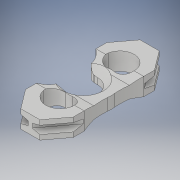
# Autodesk Inventor part: Attempted redesign Andrew.8.Offcentered.LargerAccesss
Saved by Autodesk Inventor 2017 (Build 210142000, 142)
## iProperties
Created: 2016-03-15
Part Number: Attempted redesign Andrew.8.Offcentered.LargerAccesss
Material: Generic
Document SubType Name: Modeling
Designer: Opto Neuro Core
Density: 1 g/cm^3
Appearance: Default
Author: Opto Neuro Core
Autodesk Inventor part; units mm, degrees
ref_plane "YZ Plane" through (0, 0, 0) normal (1, 0, 0) x (0, 1, 0)
ref_plane "XZ Plane" through (0, 0, 0) normal (0, 1, 0) x (-1, 0, 0)
ref_plane "XY Plane" through (0, 0, 0) normal (0, 0, 1) x (1, 0, 0)
sketch "Sketch1" plane through (0, 0, 0) normal (0, 1, 0) x (-1, 0, 0)
  line L0 (0.0095, 15.8699) -> (12.7095, 15.8699) construction
  line L1 (8.8995, 15.8699) -> (12.7095, 10.7899) construction
  line L2 (3.8195, 15.8699) -> (0.0095, 10.7899) construction
  line L3 (8.8995, 15.8699) -> (3.8195, 15.8699) construction
  line L4 (0.0095, 10.7899) -> (0.0095, 7.9324) construction
  line L5 (12.7095, 10.7899) -> (12.7095, 7.9324) construction
  line L6 (12.7095, 7.9324) -> (0.0095, 7.9324) construction
  line L7 (12.7095, 7.9324) -> (0.0095, 7.9324)
  line L8 (0.0095, 7.9324) -> (0.0095, 10.7899)
  line L9 (0.0095, 10.7899) -> (3.8195, 15.8699)
  line L10 (3.8195, 15.8699) -> (8.8995, 15.8699)
  line L11 (8.8995, 15.8699) -> (12.7095, 10.7899)
  line L12 (12.7095, 10.7899) -> (12.7095, 7.9324)
  line L13 (6.3547, -0.0026) -> (-13.1747, -0.0026) construction
  line L14 (0.0095, -15.875) -> (12.7095, -15.875) construction
  line L15 (8.8995, -15.875) -> (12.7095, -10.795) construction
  line L16 (3.8195, -15.875) -> (0.0095, -10.795) construction
  line L17 (8.8995, -15.875) -> (3.8195, -15.875) construction
  line L18 (0.0095, -10.795) -> (0.0095, -7.9375) construction
  line L19 (12.7095, -10.795) -> (12.7095, -7.9375) construction
  line L20 (12.7095, -7.9375) -> (0.0095, -7.9375) construction
  line L21 (12.7095, -7.9375) -> (0.0095, -7.9375)
  line L22 (0.0095, -7.9375) -> (0.0095, -10.795)
  line L23 (0.0095, -10.795) -> (3.8195, -15.875)
  line L24 (3.8195, -15.875) -> (8.8995, -15.875)
  line L25 (8.8995, -15.875) -> (12.7095, -10.795)
  line L26 (12.7095, -10.795) -> (12.7095, -7.9375)
  point P0 (0, 0)
  dimension "d8" = 6.35
  dimension "d83" = 2.8575
  constraints: 54 end point, 8 symmetric about line, 5 collinear, 4 point on line, 3 horizontal, 2 vertical, 1 perpendicular
  measures "d8" distance of L2.start L2.end
  measures "d83" distance of L2.end L4.end
extrude "Extrusion11" add sketch "Sketch1" along normal blind 0.508
sketch "Sketch12" plane through (0, 0.508, 0) normal (0, 1, 0) x (1, 0, 0)
  line L0 (-0.0095, 10.795) -> (-3.8195, 15.875) projected
  line L1 (-3.8195, 15.875) -> (-8.8995, 15.875) projected
  line L2 (-8.8995, 15.875) -> (-12.7095, 10.795) projected
  line L3 (-12.7095, 10.795) -> (-12.7095, 7.9375) projected
  line L4 (-12.7095, 7.9375) -> (-0.0095, 7.9375) projected
  line L5 (-0.0095, 7.9375) -> (-0.0095, 10.795) projected
  line L6 (-3.8195, -15.8699) -> (-0.0095, -10.7899) projected
  line L7 (-0.0095, -10.7899) -> (-0.0095, -7.9324) projected
  line L8 (-0.0095, -7.9324) -> (-12.7095, -7.9324) projected
  line L9 (-12.7095, -7.9324) -> (-12.7095, -10.7899) projected
  line L10 (-12.7095, -10.7899) -> (-8.8995, -15.8699) projected
  line L11 (-8.8995, -15.8699) -> (-3.8195, -15.8699) projected
  point P0 (0, 0)
extrude "Extrusion12" add sketch "Sketch12" along normal blind 0.5207
chamfer "Chamfer17" distance 1.5935 distance2 0.5207 1 edges at (-1.9145, 1.0287, -13.335) measured on face at (-2.3145, 1.0287, -13.035)
chamfer "Chamfer18" distance 1.5935 distance2 0.5207 1 edges at (-10.8045, 1.0287, -13.335) measured on face at (-10.4045, 1.0287, -13.035)
chamfer "Chamfer19" distance 1.5935 distance2 0.5207 1 edges at (-1.9145, 1.0287, 13.3299) measured on face at (-2.3145, 1.0287, 13.0299)
chamfer "Chamfer20" distance 1.5935 distance2 0.5207 1 edges at (-10.8045, 1.0287, 13.3299) measured on face at (-10.4045, 1.0287, 13.0299)
sketch "Sketch14" plane through (0, 1.0287, 0) normal (0, 1, 0) x (1, 0, 0)
  line L0 (-12.7095, 8.1392) -> (-6.9076, 15.875) projected
  line L1 (-12.7095, 8.1392) -> (-12.7095, 7.9375) projected
  line L2 (-12.7095, 7.9375) -> (-0.0095, 7.9375) projected
  line L3 (-0.0095, 7.9375) -> (-0.0095, 8.1392) projected
  line L4 (-5.8113, 15.875) -> (-0.0095, 8.1392) projected
  line L5 (-5.8113, 15.875) -> (-6.9076, 15.875) projected
  line L6 (-6.9076, -15.8699) -> (-12.7095, -8.1341) projected
  line L7 (-6.9076, -15.8699) -> (-5.8113, -15.8699) projected
  line L8 (-0.0095, -8.1341) -> (-5.8113, -15.8699) projected
  line L9 (-0.0095, -8.1341) -> (-0.0095, -7.9324) projected
  line L10 (-0.0095, -7.9324) -> (-12.7095, -7.9324) projected
  line L11 (-12.7095, -7.9324) -> (-12.7095, -8.1341) projected
  point P0 (0, 0)
extrude "Extrusion13" add sketch "Sketch14" along normal blind 1.1176
sketch "Sketch15" plane through (0, 2.1463, 0) normal (0, 1, 0) x (1, 0, 0)
  line L0 (-3.8195, 15.875) -> (-0.0095, 10.795) projected
  line L1 (-0.0095, 10.795) -> (-0.0095, 7.9375) projected
  line L2 (-0.0095, 7.9375) -> (-12.7095, 7.9375) projected
  line L3 (-12.7095, 7.9375) -> (-12.7095, 10.795) projected
  line L4 (-12.7095, 10.795) -> (-8.8995, 15.875) projected
  line L5 (-8.8995, 15.875) -> (-3.8195, 15.875) projected
  line L6 (-3.8195, -15.8699) -> (-0.0095, -10.7899) projected
  line L7 (-8.8995, -15.8699) -> (-3.8195, -15.8699) projected
  line L8 (-12.7095, -10.7899) -> (-8.8995, -15.8699) projected
  line L9 (-12.7095, -7.9324) -> (-12.7095, -10.7899) projected
  line L10 (-0.0095, -7.9324) -> (-12.7095, -7.9324) projected
  line L11 (-0.0095, -10.7899) -> (-0.0095, -7.9324) projected
  point P0 (0, 0)
extrude "Extrusion14" add sketch "Sketch15" along normal blind 0.5207
sketch "Sketch16" plane through (0, 2.667, 0) normal (0, 1, 0) x (1, 0, 0)
  line L0 (-0.0095, 10.795) -> (-3.8195, 15.875) projected
  line L1 (-3.8195, 15.875) -> (-8.8995, 15.875) projected
  line L2 (-8.8995, 15.875) -> (-12.7095, 10.795) projected
  line L3 (-12.7095, 10.795) -> (-12.7095, 7.9375) projected
  line L4 (-12.7095, 7.9375) -> (-0.0095, 7.9375) projected
  line L5 (-0.0095, 7.9375) -> (-0.0095, 10.795) projected
  line L6 (-3.8195, -15.8699) -> (-0.0095, -10.7899) projected
  line L7 (-0.0095, -10.7899) -> (-0.0095, -7.9324) projected
  line L8 (-0.0095, -7.9324) -> (-12.7095, -7.9324) projected
  line L9 (-12.7095, -7.9324) -> (-12.7095, -10.7899) projected
  line L10 (-12.7095, -10.7899) -> (-8.8995, -15.8699) projected
  line L11 (-8.8995, -15.8699) -> (-3.8195, -15.8699) projected
  point P0 (0, 0)
extrude "Extrusion15" add sketch "Sketch16" along normal blind 0.508
chamfer "Chamfer21" distance 1.5935 distance2 0.5207 1 edges at (-1.9145, 2.1463, -13.335) measured on face at (-2.3145, 2.1463, -13.035)
chamfer "Chamfer22" distance 1.5935 distance2 0.5207 1 edges at (-10.8045, 2.1463, -13.335) measured on face at (-10.4045, 2.1463, -13.035)
chamfer "Chamfer23" distance 1.5935 distance2 0.5207 1 edges at (-1.9145, 2.1463, 13.3299) measured on face at (-2.3145, 2.1463, 13.0299)
chamfer "Chamfer24" distance 1.5935 distance2 0.5207 1 edges at (-10.8045, 2.1463, 13.3299) measured on face at (-10.4045, 2.1463, 13.0299)
sketch "Sketch18" plane through (0, 3.175, 0) normal (0, 1, 0) x (1, 0, 0)
  line L0 (-0.0095, 10.795) -> (-3.8195, 15.875) construction
  line L1 (-3.8195, 15.875) -> (-8.8995, 15.875) construction
  line L2 (-8.8995, 15.875) -> (-12.7095, 10.795) construction
  line L3 (-12.7095, 10.795) -> (-12.7095, 7.9375) construction
  line L4 (-12.7095, 7.9375) -> (-0.0095, 7.9375) construction
  line L5 (-0.0095, 7.9375) -> (-0.0095, 10.795) construction
  line L6 (-3.8195, -15.8699) -> (-0.0095, -10.7899) construction
  line L7 (-0.0095, -10.7899) -> (-0.0095, -7.9324) construction
  line L8 (-0.0095, -7.9324) -> (-12.7095, -7.9324) construction
  line L9 (-12.7095, -7.9324) -> (-12.7095, -10.7899) construction
  line L10 (-12.7095, -10.7899) -> (-8.8995, -15.8699) construction
  line L11 (-8.8995, -15.8699) -> (-3.8195, -15.8699) construction
  line L12 (-0.0095, 7.9375) -> (-12.7095, 7.9375) construction
  line L13 (-6.3595, 7.9375) -> (-6.3595, -7.9324) construction
  line L14 (-0.0095, 7.9375) -> (-0.0095, -7.9324) construction
  line L15 (-12.7095, 7.9375) -> (-12.7095, -7.9324) construction
  line L16 (-12.7095, 7.9375) -> (-12.7095, 10.795) construction
  line L17 (-0.0095, 9.3663) -> (-4.4274, 3.2863) construction
  line L18 (-4.4274, -3.2812) -> (-0.0095, -9.3611) construction
  line L19 (-0.0095, -10.7899) -> (-0.0095, -7.9324) construction
  line L20 (-12.7095, -8.1341) -> (-12.7095, -10.7899) construction
  line L21 (-12.7095, -9.462) -> (-8.2916, -3.2812) construction
  line L22 (-12.7095, 9.3662) -> (-8.2916, 3.2863) construction
  line L23 (-2.5495, -5.8656) -> (-2.5495, 0.0026) construction
  line L24 (-2.5495, 0.0026) -> (-2.5495, 5.8707) construction
  line L25 (-10.1695, 0.0026) -> (-10.1695, -5.9084) construction
  line L26 (-10.1695, 0.0026) -> (-10.1695, 5.8707) construction
  circle A0 centre (-6.3595, 0.0026) radius 5.715 construction
  line L27 (-0.0095, 7.9375) -> (-3.3041, 4.8322)
  line L28 (-3.3041, -4.8271) -> (-0.0095, -7.9324)
  arc A1 (-3.3041, -4.8271) -> (-3.3041, 4.8322) centre (-6.3595, 0.0026) ccw
  line L29 (-0.0095, 7.9375) -> (-12.7095, 7.9375)
  line L30 (-0.0095, -7.9324) -> (-12.7095, -7.9324)
  circle A2 centre (-9.1475, 0.0122) radius 3.81
  line L31 (11.1379, 29.9505) -> (12.3599, 29.9505)
  line L32 (-12.7095, 7.9375) -> (-12.7095, 1.3643)
  line L33 (-12.7095, -1.3399) -> (-12.7095, 1.3643)
  line L34 (-12.7095, -1.3399) -> (-12.7095, -7.9324)
  point P0 (-9.4149, 4.8322)
  point P1 (-9.4023, -4.8351)
  dimension "d119" = 11.43
  dimension "d162" = 7.62
  constraints: 38 end point, 11 point on line, 8 point on circle, 6 midpoint, 3 centre point, 3 horizontal, 2 collinear, 2 concentric, 2 parallel, 2 vertical
  measures "d119" diameter of A0
  measures "d162" diameter of A2
extrude "Extrusion16" add sketch "Sketch18" against normal blind 3.175 contours L27 A1 L28 L30 L34 A2 L32 L29
fillet "Fillet1" radius 3.175 2 edges at (-3.3041, 1.5875, 4.8271) (-3.3041, 1.5875, -4.8322)
sketch "Sketch19" plane through (0, 3.175, 0) normal (0, 1, 0) x (1, 0, 0)
  arc A0 (-1.5083, -3.0185) -> (-1.5083, 3.0237) centre (-6.3595, 0.0026) ccw construction
  line L0 (-3.8195, 15.875) -> (-8.8995, 15.875) construction
  arc A1 (-11.2107, 3.0237) -> (-11.2092, -3.0209) centre (-6.3595, 0.0026) ccw construction
  line L1 (-12.7095, 8.1392) -> (-6.9076, 15.875) construction
  line L2 (-6.9076, 15.875) -> (-12.7095, 8.1392) construction
  line L3 (-5.8113, 15.875) -> (-0.0095, 8.1392) construction
  line L4 (-0.0095, 8.1392) -> (-5.8113, 15.875) construction
  line L5 (-6.9076, -15.8699) -> (-12.7095, -8.1341) construction
  line L6 (-12.7095, -8.1341) -> (-6.9076, -15.8699) construction
  line L7 (-0.0095, -8.1341) -> (-5.8113, -15.8699) construction
  line L8 (-5.8113, -15.8699) -> (-0.0095, -8.1341) construction
  line L9 (-8.8995, 15.875) -> (-3.8195, 15.875) construction
  line L10 (-8.8995, -15.8699) -> (-3.8195, -15.8699) construction
  line L11 (-6.3595, 15.875) -> (-6.3595, -15.8699) construction
  line L12 (-6.3595, 0.0026) -> (-6.3595, 15.875) construction
  line L13 (-6.3595, 0.0026) -> (-6.3595, -15.8699) construction
  line L14 (-6.3595, -7.9337) -> (5.5565, -7.9337) construction
  line L15 (-6.3595, 7.9388) -> (8.721, 7.9388) construction
  arc A2 (-3.803, 5.1139) -> (-8.916, 5.1139) centre (-6.3595, 7.9388) ccw construction
  arc A3 (-8.916, -5.1087) -> (-3.803, -5.1087) centre (-6.3595, -7.9337) ccw construction
  circle A4 centre (-6.3595, 0.0026) radius 5.715 construction
  arc A5 (-3.803, 5.1139) -> (-8.916, 5.1139) centre (-6.3595, 7.9388) ccw
  arc A6 (-3.803, 5.1139) -> (-8.916, 5.1139) centre (-6.3595, 0.0026) ccw
  arc A7 (-8.916, -5.1087) -> (-3.803, -5.1087) centre (-6.3595, -7.9337) ccw
  arc A8 (-8.916, -5.1087) -> (-3.803, -5.1087) centre (-6.3595, 0.0026) ccw
  point P0 (0, 0)
  dimension "d123" = 7.62
  dimension "d124" = 7.62
  constraints: 16 point on circle, 10 end point, 7 centre point, 4 concentric, 4 midpoint, 3 coincident, 2 horizontal, 1 collinear, 1 perpendicular
  measures "d123" diameter of A2
  measures "d124" diameter of A3
extrude "Extrusion17" cut sketch "Sketch19" against normal blind 25.4
fillet "Fillet2" radius 2.54 4 edges at (-8.916, 1.5875, 5.1087) (-3.803, 1.5875, 5.1087) (-3.803, 1.5875, -5.1139) (-8.916, 1.5875, -5.1139)
sketch "Sketch20" plane through (0, 3.175, 0) normal (0, 1, 0) x (1, 0, 0)
  line L0 (-3.8195, -15.8699) -> (-0.0095, -10.7899) projected
  line L1 (-0.0095, -10.7899) -> (-0.0095, -7.9324) projected
  line L2 (-0.0095, -7.9324) -> (-0.9909, -7.0074) projected
  arc A0 (-1.5083, -3.0185) -> (-0.9909, -7.0074) centre (1.1868, -4.6969) ccw projected
  arc A1 (-1.5083, -3.0185) -> (-1.5083, 3.0237) centre (-6.3595, 0.0026) ccw projected
  arc A2 (-0.9909, 7.0125) -> (-1.5083, 3.0237) centre (1.1868, 4.7021) ccw projected
  line L3 (-0.9909, 7.0125) -> (-0.0095, 7.9375) projected
  line L4 (-0.0095, 7.9375) -> (-0.0095, 10.795) projected
  line L5 (-0.0095, 10.795) -> (-3.8195, 15.875) projected
  line L6 (-3.8195, 15.875) -> (-8.8995, 15.875) projected
  line L7 (-8.8995, 15.875) -> (-12.7095, 10.795) projected
  line L8 (-12.7095, 10.795) -> (-12.7095, 7.9375) projected
  line L9 (-12.7095, 7.9375) -> (-11.7281, 7.0125) projected
  arc A3 (-11.2107, 3.0237) -> (-11.7281, 7.0125) centre (-13.9058, 4.7021) ccw projected
  arc A4 (-11.2107, 3.0237) -> (-11.2092, -3.0209) centre (-6.3595, 0.0026) ccw projected
  arc A5 (-11.7332, -7.018) -> (-11.2092, -3.0209) centre (-13.9035, -4.7006) ccw projected
  line L10 (-11.7332, -7.018) -> (-12.7095, -7.9324) projected
  line L11 (-12.7095, -7.9324) -> (-12.7095, -10.7899) projected
  line L12 (-12.7095, -10.7899) -> (-8.8995, -15.8699) projected
  line L13 (-8.8995, -15.8699) -> (-3.8195, -15.8699) projected
  arc A6 (-7.225, -5.6465) -> (-5.494, -5.6465) centre (-6.3595, 0.0026) ccw projected
  arc A7 (-2.609, -8.6044) -> (-5.494, -5.6465) centre (-5.1093, -8.1572) ccw projected
  arc A8 (-10.11, -8.6044) -> (-2.609, -8.6044) centre (-6.3595, -7.9337) ccw projected
  arc A9 (-7.225, -5.6465) -> (-10.11, -8.6044) centre (-7.6097, -8.1572) ccw projected
  arc A10 (-5.494, 5.6516) -> (-7.225, 5.6516) centre (-6.3595, 0.0026) ccw projected
  arc A11 (-10.11, 8.6095) -> (-7.225, 5.6516) centre (-7.6097, 8.1624) ccw projected
  arc A12 (-2.609, 8.6095) -> (-10.11, 8.6095) centre (-6.3595, 7.9388) ccw projected
  arc A13 (-5.494, 5.6516) -> (-2.609, 8.6095) centre (-5.1093, 8.1624) ccw projected
  circle A14 centre (-6.3595, 0.0026) radius 4.7244 projected
  point P0 (0, 0)
  point P1 (-10.1695, -7.9324)
  point P2 (-2.5495, -7.9324)
  point P3 (-2.5495, 7.9375)
  point P4 (-10.1695, 7.9375)
extrude "Extrusion18" add sketch "Sketch20" along normal blind 0.762
sketch "Sketch21" plane through (0, 0, 0) normal (0, -1, 0) x (1, 0, 0)
  arc A0 (-7.225, -5.6516) -> (-5.494, -5.6516) centre (-6.3595, -0.0026) ccw projected
  arc A1 (-2.609, -8.6095) -> (-5.494, -5.6516) centre (-5.1093, -8.1624) ccw projected
  arc A2 (-10.11, -8.6095) -> (-2.609, -8.6095) centre (-6.3595, -7.9388) ccw projected
  arc A3 (-7.225, -5.6516) -> (-10.11, -8.6095) centre (-7.6097, -8.1624) ccw projected
  arc A4 (-5.494, 5.6465) -> (-7.225, 5.6465) centre (-6.3595, -0.0026) ccw projected
  arc A5 (-10.11, 8.6044) -> (-7.225, 5.6465) centre (-7.6097, 8.1572) ccw projected
  arc A6 (-2.609, 8.6044) -> (-10.11, 8.6044) centre (-6.3595, 7.9337) ccw projected
  arc A7 (-5.494, 5.6465) -> (-2.609, 8.6044) centre (-5.1093, 8.1572) ccw projected
  circle A8 centre (-6.3595, -0.0026) radius 3.81 projected
  line L0 (-3.8195, 15.8699) -> (-0.0095, 10.7899) projected
  line L1 (-8.8995, 15.8699) -> (-3.8195, 15.8699) projected
  line L2 (-12.7095, 10.7899) -> (-8.8995, 15.8699) projected
  line L3 (-12.7095, 7.9324) -> (-12.7095, 10.7899) projected
  line L4 (-12.7095, 7.9324) -> (-11.7332, 7.018) projected
  arc A9 (-11.2092, 3.0209) -> (-11.7332, 7.018) centre (-13.9035, 4.7006) ccw projected
  arc A10 (-11.2092, 3.0209) -> (-11.2107, -3.0237) centre (-6.3595, -0.0026) ccw projected
  arc A11 (-11.7281, -7.0125) -> (-11.2107, -3.0237) centre (-13.9058, -4.7021) ccw projected
  line L5 (-11.7281, -7.0125) -> (-12.7095, -7.9375) projected
  line L6 (-12.7095, -7.9375) -> (-12.7095, -10.795) projected
  line L7 (-12.7095, -10.795) -> (-8.8995, -15.875) projected
  line L8 (-8.8995, -15.875) -> (-3.8195, -15.875) projected
  line L9 (-3.8195, -15.875) -> (-0.0095, -10.795) projected
  line L10 (-0.0095, -10.795) -> (-0.0095, -7.9375) projected
  line L11 (-0.0095, -7.9375) -> (-0.9909, -7.0125) projected
  arc A12 (-1.5083, -3.0237) -> (-0.9909, -7.0125) centre (1.1868, -4.7021) ccw projected
  arc A13 (-1.5083, -3.0237) -> (-1.5083, 3.0185) centre (-6.3595, -0.0026) ccw projected
  arc A14 (-0.9909, 7.0074) -> (-1.5083, 3.0185) centre (1.1868, 4.6969) ccw projected
  line L12 (-0.9909, 7.0074) -> (-0.0095, 7.9324) projected
  line L13 (-0.0095, 10.7899) -> (-0.0095, 7.9324) projected
  point P0 (0, 0)
  point P1 (-10.1695, -7.9375)
  point P2 (-2.5495, -7.9375)
  point P3 (-2.5495, 7.9324)
  point P4 (-10.1695, 7.9324)
extrude "Extrusion19" add sketch "Sketch21" along normal blind 0.762
sketch "Sketch24" plane through (-12.7095, 1.0287, -8.1392) normal (-1, 0, 0) x (0, 0, 1)
  line L0 (0.2017, 2.9083) -> (0.2017, -1.7907) construction
  line L1 (18.9291, 1.6383) -> (16.2733, 1.1176) construction
  line L2 (18.9291, 1.6383) -> (18.9291, 2.9083) construction
  line L3 (16.0716, 2.9083) -> (18.9291, 2.9083) construction
  line L4 (16.0716, 2.1463) -> (16.0716, 2.9083) construction
  line L5 (18.9291, -1.7907) -> (16.0716, -1.7907) construction
  line L6 (18.9291, -1.7907) -> (18.9291, -0.5207) construction
  line L7 (16.2733, 0) -> (18.9291, -0.5207) construction
  line L8 (16.2733, 0) -> (16.2733, 1.1176) construction
  line L9 (3.4122, 2.9083) -> (12.861, 2.9083) construction
  line L10 (5.1155, -1.7907) -> (1.1267, -1.7907) construction
  line L11 (3.4122, -1.7907) -> (3.4122, -1.0287) construction
  line L12 (3.4122, -1.7907) -> (4.1742, -1.7907) construction
  line L13 (12.861, -1.7907) -> (12.861, -1.0287) construction
  line L14 (12.861, -1.7907) -> (13.623, -1.7907) construction
  line L15 (12.861, 2.1463) -> (16.0716, 2.9083)
  line L16 (16.0716, 2.9083) -> (0.2017, 2.9083)
  line L17 (0.2017, 2.9083) -> (0.2017, -1.7907) projected
  line L18 (0.2017, -1.7907) -> (3.4122, -1.0287)
  line L19 (3.4122, -1.0287) -> (12.861, -1.0287)
  line L20 (12.861, -1.0287) -> (16.0716, -1.7907)
  line L21 (16.0716, -1.7907) -> (16.0716, 2.9083) projected
  line L22 (16.0716, -1.7907) -> (0.2017, -1.7907)
  line L23 (12.861, 2.1463) -> (3.4122, 2.1463) projected
  line L24 (3.4122, 2.1463) -> (0.2017, 2.9083)
  line L25 (12.861, 2.1463) -> (3.4122, 2.1463)
  line L26 (16.0716, -1.0287) -> (16.0716, -1.7907) projected
  line L27 (9.4791, 2.1463) -> (16.0716, 2.1463) projected
  line L28 (9.4791, 2.1463) -> (9.4791, -1.0287) projected
  line L29 (16.0716, -1.0287) -> (9.4791, -1.0287) projected
  point P0 (8.1392, -1.0287)
  dimension "d150" = 0.762
  dimension "d151" = 90
  dimension "d152" = 0.762
  dimension "d153" = 90
  constraints: 24 end point, 6 perpendicular, 2 horizontal, 1 parallel, 1 point on line, 1 vertical
  measures "d150" distance of L11.start L11.end
  measures "d151" angle of L12 L11
  measures "d152" distance of L13.start L13.end
  measures "d153" angle of L14 L13
extrude "Extrusion22" cut sketch "Sketch24" against normal through all contours L23 L24 L16 L15 | L19 L20 L22 L18
sketch "Sketch29" plane through (0, 3.175, 0) normal (0, 1, 0) x (1, 0, 0)
  arc A0 (-10.7309, 4.727) -> (-9.2176, 3.8215) centre (-8.8686, 6.1221) ccw
  line L0 (-9.2176, 3.8215) -> (-9.2176, -3.7972)
  arc A1 (-10.7309, 4.727) -> (-11.7281, 7.0125) centre (-13.9058, 4.7021) ccw projected
  line L1 (-11.7281, 7.0125) -> (-12.7095, 7.9375) projected
  arc A2 (-11.7332, -7.018) -> (-10.7286, -4.7218) centre (-13.9035, -4.7006) ccw projected
  line L2 (-12.7095, -7.9324) -> (-11.7332, -7.018) projected
  line L3 (-14.5036, 7.9375) -> (-13.8471, -7.9793)
  line L4 (-13.8471, -7.9793) -> (-12.7095, -7.9324)
  line L5 (-11.7281, 7.0125) -> (-12.7095, 7.9375) projected
  line L6 (-12.7095, 7.9375) -> (-14.5036, 7.9375)
  arc A3 (-10.7309, 4.727) -> (-11.7281, 7.0125) centre (-13.9058, 4.7021) ccw
  line L7 (-11.7281, 7.0125) -> (-12.7095, 7.9375)
  arc A4 (-9.2176, -3.7972) -> (-10.7286, -4.7218) centre (-8.7916, -6.1901) ccw
  point P0 (0, 0)
  constraints: 10 end point, 6 point on circle, 3 centre point, 1 horizontal, 1 perpendicular, 1 vertical
extrude "Extrusion25" cut sketch "Sketch29" against normal blind 25.4
sketch "Sketch30" plane through (0, 3.937, 0) normal (0, 1, 0) x (1, 0, 0)
  arc A0 (-9.2176, -3.7972) -> (-10.7286, -4.7218) centre (-8.7916, -6.1901) ccw projected
  line L0 (-10.7286, -4.7218) -> (-1.9881, -4.7218) projected
  arc A1 (-1.5083, -3.0185) -> (-1.9881, -4.7218) centre (1.1868, -4.6969) ccw projected
  arc A2 (-1.5083, -3.0185) -> (-1.5083, 3.0237) centre (-6.3595, 0.0026) ccw construction
  arc A3 (-1.9881, 4.727) -> (-1.5083, 3.0237) centre (1.1868, 4.7021) ccw projected
  line L1 (-10.7309, 4.727) -> (-1.9881, 4.727) projected
  arc A4 (-10.7309, 4.727) -> (-9.2176, 3.8215) centre (-8.8686, 6.1221) ccw construction
  arc A5 (-9.2176, -3.7972) -> (-9.2176, 3.8215) centre (-9.1475, 0.0122) ccw construction
  line L2 (-0.6445, 0.0026) -> (-1.6605, 0.0026) construction
  arc A6 (-8.1337, -3.7972) -> (-8.1337, 3.8215) centre (-8.1337, 0.0122) ccw construction
  line L3 (-8.1337, -3.7972) -> (-9.2176, -3.7972)
  arc A7 (-10.7309, 4.727) -> (-9.2176, 3.8215) centre (-8.8686, 6.1221) ccw construction
  line L4 (-9.2176, 3.8215) -> (-8.1337, 3.8215) construction
  line L5 (-8.1337, 3.8215) -> (-9.2176, 3.8215) construction
  arc A8 (-8.1337, -3.7972) -> (-8.1337, 3.8215) centre (-8.1337, 0.0122) ccw
  arc A9 (-9.2176, -3.7972) -> (-9.2176, 3.8215) centre (-9.1475, 0.0122) ccw construction
  line L6 (-9.2176, 3.8215) -> (-9.2176, -3.7972) construction
  line L7 (-9.2176, -3.7972) -> (-9.2176, 3.8215)
  line L8 (-9.2176, 3.8215) -> (-8.1337, 3.8215)
  dimension "d175" = 1.016
  constraints: 14 end point, 6 point on circle, 3 horizontal, 2 centre point, 2 collinear, 1 coincident, 1 tangent, 1 vertical
  measures "d175" distance of L2.start L2.end
extrude "Extrusion26" cut sketch "Sketch30" against normal blind 25.4
sketch "Sketch31" plane through (0, 0, 0) normal (0, 0, 1) x (1, 0, 0)
  ellipse E0 centre (-6.3595, 2.0537) end of major axis (-0.6445, 2.0537) minor radius 1.3564 (-5.494, 3.3945) -> (-7.225, 3.3945) ccw construction
  line L0 (-5.494, -0.2195) -> (-5.494, 3.3945) construction
  ellipse E1 centre (-6.3595, 1.1213) end of major axis (-12.0745, 1.1213) minor radius 1.3564 (-7.225, -0.2195) -> (-5.494, -0.2195) ccw construction
  line L1 (-7.225, 3.3945) -> (-7.225, -0.2195) construction
  line L2 (-6.3595, 1.1213) -> (-6.3595, 7.232) construction
  line L3 (-9.0774, 3.175) -> (-8.1337, 3.175) construction
  line L4 (-8.1337, 3.175) -> (-8.1337, 3.175) construction
  line L5 (-8.1337, 3.175) -> (-9.0774, 3.175) construction
  line L6 (-9.0774, 3.175) -> (-9.2176, 3.175) construction
  line L7 (-9.2176, 3.175) -> (-10.7286, 3.175) construction
  line L8 (-10.7286, 3.175) -> (-1.9881, 3.175) construction
  line L9 (-1.5083, 3.175) -> (-1.9881, 3.175) construction
  line L10 (-1.5083, 3.175) -> (-1.5083, 3.175) construction
  line L11 (-1.9881, 3.175) -> (-1.5083, 3.175) construction
  line L12 (-10.7309, 3.175) -> (-1.9881, 3.175) construction
  line L13 (-10.7309, 3.175) -> (-9.2176, 3.175) construction
  line L14 (-9.2176, 3.175) -> (-9.0774, 3.175) construction
  line L15 (-8.1337, 3.175) -> (-4.3244, 3.175) construction
  line L16 (-4.5852, 3.175) -> (-4.5852, 0) construction
  line L17 (-4.5852, 3.175) -> (-4.5852, 0) construction
  line L18 (-4.5852, 3.175) -> (-4.5852, 0) construction
  line L19 (-4.5852, 3.175) -> (-4.5852, 0) construction
  line L20 (-4.5852, 3.175) -> (-6.3595, 3.175) construction
  line L21 (-6.3595, 3.175) -> (-6.3595, 1.1213)
  line L22 (-4.5852, 3.175) -> (-2.4262, 3.175) construction
  line L23 (-10.7286, 3.175) -> (-1.9881, 3.175) construction
  line L24 (-6.3595, 1.1213) -> (-6.3595, -0.4027)
  line L25 (-8.1337, 3.175) -> (-8.1337, -3.0889)
  line L26 (-6.3595, 3.175) -> (-6.3595, 4.6761)
  line L27 (-6.3595, 4.6761) -> (0.6126, 4.6761)
  line L28 (-0.7759, 4.6761) -> (-1.0299, 4.6761)
  line L29 (-1.0299, 4.6761) -> (-1.2839, 4.6761)
  line L30 (-1.2839, 4.6761) -> (-6.3595, -0.4027)
  point P0 (0, 0)
  dimension "d179" = 1.524
  dimension "d182" = 0.254
  dimension "d183" = 0.254
  constraints: 30 end point, 6 point on line, 4 symmetric about line, 3 vertical, 1 horizontal, 1 perpendicular, 4 other
  measures "d179" distance of L2.start L24.end
  measures "d182" distance of L28.start L28.end
  measures "d183" distance of L28.end L29.end
revolve "Revolution1" cut sketch "Sketch31" angle 360 about axis through (-8.1337, 3.175, 0) along (0, -1, 0)
sketch "Sketch32" plane through (0, 3.937, 0) normal (0, 1, 0) x (1, 0, 0)
  line L0 (-10.1397, -7.9324) -> (-12.7095, -7.9324) projected
  line L1 (-12.7095, -7.9324) -> (-12.7095, -10.7899) projected
  line L2 (-12.7095, -10.7899) -> (-8.8995, -15.8699) projected
  line L3 (-8.8995, -15.8699) -> (-3.8195, -15.8699) projected
  line L4 (-3.8195, -15.8699) -> (-0.0095, -10.7899) projected
  line L5 (-0.0095, -10.7899) -> (-0.0095, -7.9324) projected
  line L6 (-0.0095, -7.9324) -> (-2.5793, -7.9324) projected
  arc A0 (-2.609, -8.6044) -> (-2.5793, -7.9324) centre (-5.1093, -8.1572) ccw projected
  arc A1 (-10.11, -8.6044) -> (-2.609, -8.6044) centre (-6.3595, -7.9337) ccw projected
  arc A2 (-10.1397, -7.9324) -> (-10.11, -8.6044) centre (-7.6097, -8.1572) ccw projected
  ellipse E0 centre (-8.1337, -1.0631) end of major axis (-8.1337, 3.4188) minor radius 4.3539 (-10.6483, -4.7218) -> (-5.6192, -4.7218) ccw projected
  line L7 (-10.7286, -4.7218) -> (-10.6483, -4.7218) projected
  arc A3 (-11.7332, -7.018) -> (-10.7286, -4.7218) centre (-13.9035, -4.7006) ccw projected
  line L8 (-12.7095, -7.9324) -> (-11.7332, -7.018) projected
  line L9 (-10.1397, -7.9324) -> (-12.7095, -7.9324) projected
  arc A4 (-7.225, -5.6465) -> (-10.1397, -7.9324) centre (-7.6097, -8.1572) ccw projected
  arc A5 (-7.225, -5.6465) -> (-5.494, -5.6465) centre (-6.3595, 0.0026) ccw projected
  arc A6 (-2.5793, -7.9324) -> (-5.494, -5.6465) centre (-5.1093, -8.1572) ccw projected
  line L10 (-0.0095, -7.9324) -> (-2.5793, -7.9324) projected
  line L11 (-0.9909, -7.0074) -> (-0.0095, -7.9324) projected
  arc A7 (-1.9881, -4.7218) -> (-0.9909, -7.0074) centre (1.1868, -4.6969) ccw projected
  line L12 (-5.6192, -4.7218) -> (-1.9881, -4.7218) projected
  arc A8 (-5.6192, -4.7218) -> (-5.6288, 4.727) centre (-8.1337, 0) ccw projected
  line L13 (-5.6192, -4.7218) -> (-1.9881, -4.7218) projected
  arc A9 (-1.5083, -3.0185) -> (-1.9881, -4.7218) centre (1.1868, -4.6969) ccw projected
  arc A10 (-1.5083, -3.0185) -> (-1.5083, 3.0237) centre (-6.3595, 0.0026) ccw projected
  arc A11 (-1.9881, 4.727) -> (-1.5083, 3.0237) centre (1.1868, 4.7021) ccw projected
  line L14 (-5.6288, 4.727) -> (-1.9881, 4.727) projected
  ellipse E1 centre (-8.1337, 1.0627) end of major axis (-8.1337, 5.5433) minor radius 4.3527 (-5.6288, 4.727) -> (-10.6387, 4.727) ccw projected
  line L15 (-5.6288, 4.727) -> (-1.9881, 4.727) projected
  arc A12 (-0.9909, 7.0125) -> (-1.9881, 4.727) centre (1.1868, 4.7021) ccw projected
  line L16 (-0.0095, 7.9375) -> (-0.9909, 7.0125) projected
  line L17 (-2.5793, 7.9375) -> (-0.0095, 7.9375) projected
  arc A13 (-5.494, 5.6516) -> (-2.5793, 7.9375) centre (-5.1093, 8.1624) ccw projected
  arc A14 (-5.494, 5.6516) -> (-7.225, 5.6516) centre (-6.3595, 0.0026) ccw projected
  arc A15 (-10.1397, 7.9375) -> (-7.225, 5.6516) centre (-7.6097, 8.1624) ccw projected
  line L18 (-12.7095, 7.9375) -> (-10.1397, 7.9375) projected
  line L19 (-11.7281, 7.0125) -> (-12.7095, 7.9375) projected
  arc A16 (-10.7309, 4.727) -> (-11.7281, 7.0125) centre (-13.9058, 4.7021) ccw projected
  line L20 (-10.7309, 4.727) -> (-10.6387, 4.727) projected
  arc A17 (-0.7229, -0.9409) -> (-0.0095, -7.9324) centre (20.9193, -2.2646) ccw
  line L21 (-1.1496, 0.0026) -> (-1.8693, 0.0026)
  arc A18 (-0.0095, 7.9375) -> (-0.7229, 0.946) centre (20.9193, 2.2698) ccw
  arc A19 (-1.5083, -3.0185) -> (-0.9909, -7.0074) centre (1.1868, -4.6969) ccw
  arc A20 (-1.5083, -3.0185) -> (-3.1437, -4.7218) centre (-6.3595, 0.0026) ccw
  line L22 (-0.9909, -7.0074) -> (-0.0095, -7.9324) projected
  line L23 (-0.0095, -7.9324) -> (-0.9909, -7.0074)
  line L24 (-0.0095, 10.795) -> (-0.0095, 7.9375)
  line L25 (-0.0095, 7.9375) -> (-2.5793, 7.9375)
  line L26 (-0.0095, 7.9375) -> (-2.5793, 7.9375)
  line L27 (-0.9909, 7.0125) -> (-0.0095, 7.9375)
  arc A21 (-0.9909, 7.0125) -> (-1.9881, 4.727) centre (1.1868, 4.7021) ccw
  line L28 (-5.6192, 4.727) -> (-1.9881, 4.727)
  line L29 (-5.6192, 4.727) -> (-1.9881, 4.727)
  arc A22 (-1.9881, 4.727) -> (-1.5083, 3.0237) centre (1.1868, 4.7021) ccw
  arc A23 (-1.5083, -3.0185) -> (-1.5083, 3.0237) centre (-6.3595, 0.0026) ccw
  arc A24 (-0.0095, 7.9375) -> (-0.7229, 0.946) centre (20.9193, 2.2698) ccw
  arc A25 (-0.9909, 7.0125) -> (-1.5083, 3.0237) centre (1.1868, 4.7021) ccw
  arc A26 (-3.1437, 4.727) -> (-1.5083, 3.0237) centre (-6.3595, 0.0026) ccw
  line L30 (-0.9909, 7.0125) -> (-0.0095, 7.9375)
  line L31 (-0.0095, 7.9375) -> (-0.9909, 7.0125)
  constraints: 25 point on circle, 20 end point, 19 symmetric about line, 10 centre point, 3 coincident, 2 point on line, 1 collinear, 1 horizontal, 9 other
extrude "Extrusion27" add sketch "Sketch32" against normal blind 4.699 contours L11 A7 A9 A10 A17 | A10 A11 A12 L16 A18
sketch "Sketch33" plane through (-12.7095, 1.0287, 8.1341) normal (-1, 0, 0) x (0, 0, 1)
  line L0 (-0.2017, -1.7907) -> (-1.1267, -1.5712) projected
  line L1 (-1.1267, -1.5712) -> (-1.1267, -1.7907) projected
  line L2 (-0.2017, -1.7907) -> (-1.1267, -1.7907) projected
  line L3 (-3.4122, -1.0287) -> (-5.1155, -1.0287) projected
  line L4 (-5.1155, -1.0287) -> (-5.1155, -1.7907) projected
  line L5 (-1.1267, -1.7907) -> (-5.1155, -1.7907) projected
  line L6 (-1.1267, -1.5712) -> (-1.1267, -1.7907) projected
  line L7 (-1.1267, -1.5712) -> (-3.4122, -1.0287) projected
  line L8 (-5.1155, -1.0287) -> (-7.1932, -1.0287) projected
  line L9 (-7.1932, -1.0287) -> (-7.1932, -1.7907) projected
  line L10 (-5.1155, -1.7907) -> (-7.1932, -1.7907) projected
  line L11 (-5.1155, -1.0287) -> (-5.1155, -1.7907) projected
  line L12 (-9.0801, -1.0287) -> (-11.1577, -1.0287) projected
  line L13 (-11.1577, -1.0287) -> (-11.1577, -1.7907) projected
  line L14 (-9.0801, -1.7907) -> (-11.1577, -1.7907) projected
  line L15 (-9.0801, -1.0287) -> (-9.0801, -1.7907) projected
  line L16 (-11.1577, -1.0287) -> (-12.861, -1.0287) projected
  line L17 (-12.861, -1.0287) -> (-15.1466, -1.5712) projected
  line L18 (-15.1466, -1.5712) -> (-15.1466, -1.7907) projected
  line L19 (-11.1577, -1.7907) -> (-15.1466, -1.7907) projected
  line L20 (-11.1577, -1.0287) -> (-11.1577, -1.7907) projected
  line L21 (-15.1466, -1.5712) -> (-16.0716, -1.7907) projected
  line L22 (-15.1466, -1.7907) -> (-16.0716, -1.7907) projected
  line L23 (-15.1466, -1.5712) -> (-15.1466, -1.7907) projected
  line L24 (-16.0716, 2.9083) -> (-15.1466, 2.6888) projected
  line L25 (-15.1466, 2.9083) -> (-15.1466, 2.6888) projected
  line L26 (-16.0716, 2.9083) -> (-15.1466, 2.9083) projected
  line L27 (-12.861, 2.1463) -> (-11.1577, 2.1463) projected
  line L28 (-11.1577, 2.9083) -> (-11.1577, 2.1463) projected
  line L29 (-15.1466, 2.9083) -> (-11.1577, 2.9083) projected
  line L30 (-15.1466, 2.9083) -> (-15.1466, 2.6888) projected
  line L31 (-15.1466, 2.6888) -> (-12.861, 2.1463) projected
  line L32 (-11.1577, 2.1463) -> (-9.0801, 2.1463) projected
  line L33 (-9.0801, 2.9083) -> (-9.0801, 2.1463) projected
  line L34 (-11.1577, 2.9083) -> (-9.0801, 2.9083) projected
  line L35 (-11.1577, 2.9083) -> (-11.1577, 2.1463) projected
  line L36 (-7.1932, 2.1463) -> (-5.1155, 2.1463) projected
  line L37 (-5.1155, 2.9083) -> (-5.1155, 2.1463) projected
  line L38 (-7.1932, 2.9083) -> (-5.1155, 2.9083) projected
  line L39 (-7.1932, 2.9083) -> (-7.1932, 2.1463) projected
  line L40 (-5.1155, 2.1463) -> (-3.4122, 2.1463) projected
  line L41 (-3.4122, 2.1463) -> (-1.1267, 2.6888) projected
  line L42 (-1.1267, 2.9083) -> (-1.1267, 2.6888) projected
  line L43 (-5.1155, 2.9083) -> (-1.1267, 2.9083) projected
  line L44 (-5.1155, 2.9083) -> (-5.1155, 2.1463) projected
  line L45 (-1.1267, 2.6888) -> (-0.2017, 2.9083) projected
  line L46 (-1.1267, 2.9083) -> (-0.2017, 2.9083) projected
  line L47 (-1.1267, 2.9083) -> (-1.1267, 2.6888) projected
  point P0 (-8.1341, -1.0287)
extrude "Extrusion28" cut sketch "Sketch33" against normal blind 25.4
body "Solid2"
